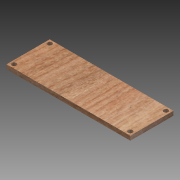
# Autodesk Inventor part: Plade
Saved by Autodesk Inventor 2012 (Build 160160000, 160)
## iProperties
Created: 2012-02-28
Part Number: Plade
Material: Default
Document SubType Name: Modeling
Designer: Grailas
Density: 1 g/cm^3
Author: Grailas
Autodesk Inventor part; units mm, degrees
ref_plane "YZ Plane" through (0, 0, 0) normal (1, 0, 0) x (0, 1, 0)
ref_plane "XZ Plane" through (0, 0, 0) normal (0, 1, 0) x (-1, 0, 0)
ref_plane "XY Plane" through (0, 0, 0) normal (0, 0, 1) x (1, 0, 0)
sketch "Sketch1" plane through (0, 0, 0) normal (0, 0, 1) x (1, 0, 0)
  line L0 (-107.5, 37.5) -> (107.5, 37.5)
  line L1 (107.5, 37.5) -> (107.5, -37.5)
  line L2 (107.5, -37.5) -> (-107.5, -37.5)
  line L3 (-107.5, -37.5) -> (-107.5, 37.5)
  circle A0 centre (-101, 31) radius 4
  circle A1 centre (101, 31) radius 4
  circle A2 centre (101, -31) radius 4
  circle A3 centre (-101, -31) radius 4
  point P0 (0, 0)
  point P1 (-107.5, 0)
  point P2 (0, -37.5)
  dimension "d0" = 215
  dimension "d1" = 75
  dimension "d2" = 8
  dimension "d3" = 6.5
  dimension "d4" = 6.5
  dimension "d5" = 6.5
  dimension "d6" = 6.5
  dimension "d7" = 6.5
  dimension "d8" = 6.5
  dimension "d9" = 6.5
  dimension "d10" = 6.5
  constraints: 8 end point, 4 centre point, 3 equal radius, 2 midpoint, 2 parallel, 1 horizontal, 1 horizontal alignment, 1 perpendicular, 1 vertical alignment
  measures "d0" distance of L0.start L0.end
  measures "d1" distance of L2.end L0.start
  measures "d2" diameter of A0
  measures "d3" distance from line of L0 A0.centre
  measures "d4" distance from line of L3 A0.centre
  measures "d5" distance from line of L0 A1.centre
  measures "d6" distance from line of L1 A1.centre
  measures "d7" distance from line of L1 A2.centre
  measures "d8" distance from line of L2 A2.centre
  measures "d9" distance from line of L2 A3.centre
  measures "d10" distance from line of L3 A3.centre
extrude "Extrusion1" add sketch "Sketch1" against normal blind 7.5
equation "\"d4\" = d3"
equation "\"d5\" = d3"
equation "\"d6\" = d5"
equation "\"d7\" = d6"
equation "\"d8\" = d7"
equation "\"d9\" = d8"
equation "\"d10\" = d9"
body "Solid1"
